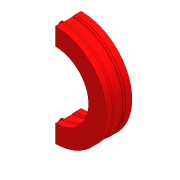
# Autodesk Inventor part: Sbend100_0
Saved by Autodesk Inventor 2022.2 (Build 262287010, 287A)
## iProperties
RuleStatus: InUse
Created: 2021-06-15
Part Number: Sbend100_0
Material: Generic
Document SubType Name: Modeling
Designer: Josep
Mass: 90127.1 g
Surface Area: 52615.5 cm^2
Volume: 90127.1 cm^3
Density: 1 g/cm^3
Appearance: SBend
Author: Josep
Autodesk Inventor part; units mm, degrees
ref_plane "YZ Plane" through (0, 0, 0) normal (1, 0, 0) x (0, 1, 0)
ref_plane "XY Plane" through (0, 0, 0) normal (0, 0, 1) x (1, 0, 0)
sketch "Sketch1" plane through (0, 0, 0) normal (0, 0, 1) x (0, 1, 0)
  line L0 (-152.5, -105) -> (152.5, -105)
  line L1 (152.5, -105) -> (152.5, 105)
  line L2 (152.5, 105) -> (-152.5, 105)
  line L3 (-152.5, 105) -> (-152.5, -105)
  line L4 (-152.5, -105) -> (152.5, 105) construction
  line L5 (152.5, -105) -> (-152.5, 105) construction
  line L6 (112.8, 66.7) -> (-112.8, 66.7)
  line L7 (-112.8, 66.7) -> (-112.8, 38.3)
  line L8 (-112.8, 38.3) -> (-20, 38.3)
  line L9 (-20, 38.3) -> (-20, -38.3)
  line L10 (-20, -38.3) -> (-112.8, -38.3)
  line L11 (-112.8, -38.3) -> (-112.8, -66.7)
  line L12 (-112.8, -66.7) -> (112.8, -66.7)
  line L13 (112.8, -66.7) -> (112.8, -38.3)
  line L14 (112.8, -38.3) -> (20, -38.3)
  line L15 (20, -38.3) -> (20, 38.3)
  line L16 (20, 38.3) -> (112.8, 38.3)
  line L17 (112.8, 38.3) -> (112.8, 66.7)
  line L18 (-80, 105) -> (80, 105)
  line L19 (80, 105) -> (80, 102.5)
  line L20 (80, 102.5) -> (-80, 102.5)
  line L21 (-80, 102.5) -> (-80, 105)
  line L22 (-52, 102.5) -> (52, 102.5)
  line L23 (52, 102.5) -> (52, 97.5)
  line L24 (52, 97.5) -> (-52, 97.5)
  line L25 (-52, 97.5) -> (-52, 102.5)
  line L26 (-80, -102.5) -> (80, -102.5)
  line L27 (80, -102.5) -> (80, -105)
  line L28 (80, -105) -> (-80, -105)
  line L29 (-80, -105) -> (-80, -102.5)
  line L30 (-52, -97.5) -> (52, -97.5)
  line L31 (52, -97.5) -> (52, -102.5)
  line L32 (52, -102.5) -> (-52, -102.5)
  line L33 (-52, -102.5) -> (-52, -97.5)
  point P0 (0, 0)
  point P1 (20, 0)
  point P2 (-20, 0)
  point P3 (0, 0)
  point P4 (0, 66.7)
  point P5 (0, 0)
  point P6 (0, -66.7)
  point P7 (0, 102.5)
  point P8 (0, 105)
  point P9 (0, -102.5)
  point P10 (0, -105)
  dimension "d6" = 305
  dimension "d7" = 210
  dimension "d8" = 225.6
  dimension "d9" = 28.4
  dimension "d10" = 40
  dimension "d11" = 76.6
  dimension "d12" = 38.3
  dimension "d46" = 2.5
  dimension "d47" = 5
  dimension "d48" = 104
  dimension "d49" = 160
  constraints: 68 end point, 16 midpoint, 13 parallel, 9 equal length, 8 perpendicular, 6 horizontal, 3 point on line, 2 horizontal alignment, 2 vertical alignment
  measures "d6" distance of L2.end L1.end
  measures "d7" distance of L1.end L0.end
  measures "d8" distance of L6.start L6.end
  measures "d9" distance of L16.end L6.start
  measures "d10" distance between parallel lines of L9 L15
  measures "d11" distance of L14.end L15.end
  measures "d12" distance between parallel lines of L6 L2
  measures "d46" distance of L20.end L18.start
  measures "d47" distance of L24.end L22.start
  measures "d48" distance of L23.end L24.end
  measures "d49" distance of L19.end L20.end
sketch "Sketch2" plane through (0, 0, 0) normal (0, 1, 0) x (-1, 0, 0)
  line L0 (0, -700) -> (0, 700) projected
  arc A0 (499.6018, 499.9998) -> (499.6018, -499.9998) centre (500, 0) ccw
  line L1 (500, 0) -> (0, 0) construction
  line L2 (499.6018, 499.9998) -> (500, 0) construction
  line L3 (499.6018, -499.9998) -> (500, 0) construction
  dimension "d54" = 90
  dimension "d58" = 1570
  dimension "d59" = 179.909
  constraints: 6 end point, 3 point on circle, 1 centre point
  measures "d54" angle of L0 L1
  measures "d59" angle of L3 L2
sweep "Sweep1" add profiles "Sketch1" path "Sketch2" path curves A0 contours L3 L2 L21 L20 L25 L24 L23 L19 L1 L0 L27 L26 L31 L30 L33 L29
sketch "Sketch3" plane through (0, 0, 0) normal (0, 0, 1) x (0, 1, 0)
  line L0 (20, 38.3) -> (112.8, 38.3) projected
  line L1 (112.8, 38.3) -> (112.8, 66.7) projected
  line L2 (112.8, 66.7) -> (-112.8, 66.7) projected
  line L3 (-112.8, 66.7) -> (-112.8, 38.3) projected
  line L4 (-112.8, 38.3) -> (-20, 38.3) projected
  line L5 (-20, 38.3) -> (-20, -38.3) projected
  line L6 (-20, -38.3) -> (-112.8, -38.3) projected
  line L7 (-112.8, -38.3) -> (-112.8, -66.7) projected
  line L8 (-112.8, -66.7) -> (112.8, -66.7) projected
  line L9 (112.8, -66.7) -> (112.8, -38.3) projected
  line L10 (112.8, -38.3) -> (20, -38.3) projected
  line L11 (20, -38.3) -> (20, 38.3) projected
  line L12 (80, 102.5) -> (80, 105) projected
  line L13 (80, 105) -> (152.5, 105) projected
  line L14 (152.5, 105) -> (152.5, -105) projected
  line L15 (152.5, -105) -> (80, -105) projected
  line L16 (80, -105) -> (80, -102.5) projected
  line L17 (80, -102.5) -> (52, -102.5) projected
  line L18 (52, -102.5) -> (52, -97.5) projected
  line L19 (52, -97.5) -> (-52, -97.5) projected
  line L20 (-52, -97.5) -> (-52, -102.5) projected
  line L21 (-52, -102.5) -> (-80, -102.5) projected
  line L22 (-80, -102.5) -> (-80, -105) projected
  line L23 (-80, -105) -> (-152.5, -105) projected
  line L24 (-152.5, -105) -> (-152.5, 105) projected
  line L25 (-152.5, 105) -> (-80, 105) projected
  line L26 (-80, 105) -> (-80, 102.5) projected
  line L27 (-80, 102.5) -> (-52, 102.5) projected
  line L28 (-52, 102.5) -> (-52, 97.5) projected
  line L29 (-52, 97.5) -> (52, 97.5) projected
  line L30 (52, 97.5) -> (52, 102.5) projected
  line L31 (52, 102.5) -> (80, 102.5) projected
  line L32 (23.9, 65.45) -> (108.9, 65.45)
  line L33 (108.9, 65.45) -> (108.9, 39.55)
  line L34 (108.9, 39.55) -> (23.9, 39.55)
  line L35 (23.9, 39.55) -> (23.9, 65.45)
  line L36 (23.9, 65.45) -> (108.9, 39.55) construction
  line L37 (108.9, 65.45) -> (23.9, 39.55) construction
  line L38 (0, 226) -> (0, -621) projected
  line L39 (-23.9, 65.45) -> (-108.9, 65.45)
  line L40 (-108.9, 65.45) -> (-108.9, 39.55)
  line L41 (-108.9, 39.55) -> (-23.9, 39.55)
  line L42 (-23.9, 39.55) -> (-23.9, 65.45)
  point P0 (112.8, -500)
  point P1 (66.4, 52.5)
  point P2 (66.4, 52.5)
  point P3 (66.4, 38.3)
  point P4 (108.9, 52.5)
  point P5 (112.8, 52.5)
  dimension "d60" = 85
  dimension "d61" = 25.9
  constraints: 20 end point, 6 midpoint, 4 symmetric about line, 2 parallel, 1 horizontal, 1 horizontal alignment, 1 perpendicular, 1 vertical alignment
  measures "d60" distance of L33.end L34.end
  measures "d61" distance of L32.end L33.end
ref_plane "Work Plane2" through (-52.5, 66.4, 0) normal (0, 1, 0) x (-1, 0, 0)
sketch "Sketch10" plane through (-52.5, 66.4, 0) normal (0, 1, 0) x (-1, 0, 0)
  arc A0 (447.155, 433.2999) -> (447.155, -433.2999) centre (447.5, 0) ccw projected
  arc A1 (447.0487, 566.6998) -> (447.0487, -566.6998) centre (447.5, 0) ccw projected
  arc A2 (447.155, 433.2999) -> (447.0487, 566.6998) centre (447.1018, 499.9998) ccw
  arc A3 (447.0487, -566.6998) -> (447.155, -433.2999) centre (447.1018, -499.9998) ccw
  point P0 (-52.5, 0)
  constraints: 4 point on circle, 2 centre point, 2 tangent
sweep "Sweep5" [suppressed]
sketch "Sketch5" plane through (0, 0, 0) normal (0, 0, 1) x (0, 1, 0)
  line L0 (-15, 19.05) -> (15, 19.05)
  line L1 (15, 19.05) -> (15, -19.05)
  line L2 (15, -19.05) -> (-15, -19.05)
  line L3 (-15, -19.05) -> (-15, 19.05)
  line L4 (-15, 19.05) -> (15, -19.05) construction
  line L5 (15, 19.05) -> (-15, -19.05) construction
  point P0 (0, 0)
  dimension "d27" = 30
  dimension "d28" = 38.1
  constraints: 12 end point, 2 midpoint, 2 parallel, 1 horizontal, 1 perpendicular
  measures "d27" distance of L1.end L2.end
  measures "d28" distance of L0.end L1.end
sketch "Sketch6" plane through (0, 0, 0) normal (0, 1, 0) x (-1, 0, 0)
  arc A0 (499.6018, 499.9998) -> (499.6018, -499.9998) centre (500, 0) ccw projected
  line L0 (499.6018, 499.9998) -> (574.6018, 500.0596)
  line L1 (499.6018, -499.9998) -> (574.6018, -500.0596)
  dimension "d64" = 75
  dimension "d65" = 75
  constraints: 4 end point, 2 tangent
  measures "d64" distance of L0.start L0.end
  measures "d65" distance of L1.start L1.end
sweep "Sweep4" add profiles "Sketch5" path "Sketch6"
sketch "Sketch7" plane through (-574.3679, -15, 793.7782) normal (0.9999997, 0, -0.0007963) x (-0.0007963, 0, -0.9999997)
  circle A0 centre (293.7187, 15) radius 34.925
  line L0 (274.6687, 0) -> (274.6687, 30) projected
  line L1 (274.6687, 30) -> (312.7687, 30) projected
  line L2 (312.7687, 30) -> (312.7687, 0) projected
  line L3 (312.7687, 0) -> (274.6687, 0) projected
  point P0 (293.7187, 30)
  point P1 (312.7687, 15)
  dimension "d32" = 69.85
  constraints: 2 midpoint, 1 centre point, 1 horizontal alignment, 1 vertical alignment
  measures "d32" diameter of A0
extrude "Extrusion1" add sketch "Sketch7" against normal blind 12.7 contours A0 | L0 L1 L2 L3
sketch "Sketch9" plane through (-574.7964, -15, -255.7535) normal (-0.9999997, 0, -0.0007963) x (-0.0007963, 0, 0.9999997)
  circle A0 centre (-244.3061, 15) radius 34.925
  line L0 (-263.3561, 0) -> (-225.2561, 0) projected
  line L1 (-263.3561, 30) -> (-263.3561, 0) projected
  line L2 (-225.2561, 30) -> (-263.3561, 30) projected
  line L3 (-225.2561, 0) -> (-225.2561, 30) projected
  point P0 (-244.3061, 30)
  point P1 (-263.3561, 15)
  dimension "d40" = 69.85
  constraints: 2 midpoint, 1 centre point, 1 horizontal alignment, 1 vertical alignment
  measures "d40" diameter of A0
extrude "Extrusion3" add sketch "Sketch9" along normal blind 12.7 contours A0 | L1 L2 L3 L0
equation "\"d58\" = Length"
equation "\"d59\" = Angle"
equation "\"d65\" = d64"
equation "\"d40\" = d32"
equation "\"d41\" = d33"
equation "\"Angle\" = 179.909deg"
equation "\"Length\" = 1570"
equation "\"d33\" = 12.7"
body "Solid1"
body "Solid5"
